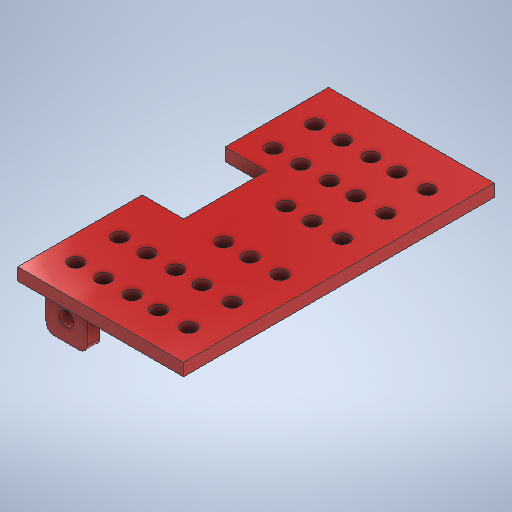
# Autodesk Inventor part: étage_servo
Saved by Autodesk Inventor 2025.1 (Build 291241000, 241)
## iProperties
Created: 2024-11-29
Part Number: étage_servo
Material: Générique
Document SubType Name: Modeling
Designer: yasmi
Density: 1 g/cm^3
Appearance: Par défaut
Author: yasmi
Autodesk Inventor part; units mm, degrees
ref_plane "YZ Plane" through (0, 0, 0) normal (1, 0, 0) x (0, 1, 0)
ref_plane "XZ Plane" through (0, 0, 0) normal (0, 1, 0) x (-1, 0, 0)
ref_plane "XY Plane" through (0, 0, 0) normal (0, 0, 1) x (1, 0, 0)
sketch "Esquisse1" plane through (0, 0, 0) normal (0, 1, 0) x (-1, 0, 0)
  line L0 (21.1354, -34.867) -> (21.1354, 40.133)
  circle A0 centre (1.447, -25.4161) radius 1.75
  circle A1 centre (1.447, -15.4161) radius 1.75
  circle A2 centre (8.3757, -15.4161) radius 1.75
  circle A3 centre (1.447, -4.8968) radius 1.75
  circle A4 centre (8.3757, -25.4161) radius 1.75
  line L1 (11.1354, 10.1032) -> (11.1354, -9.8968)
  line L2 (11.1354, -9.8968) -> (21.1354, -9.8968)
  line L3 (21.1354, -9.8968) -> (21.1354, 10.1032)
  line L4 (21.1354, 10.1032) -> (11.1354, -9.8968)
  line L5 (11.1354, 10.1032) -> (21.1354, -9.8968)
  line L6 (21.1354, 10.1032) -> (11.1354, 10.1032)
  line L7 (-18.8646, -34.867) -> (21.1354, -34.867)
  line L8 (-18.8646, -34.867) -> (21.1354, -34.867)
  line L9 (21.1354, -34.867) -> (21.1354, 40.133)
  line L10 (-18.8646, 40.133) -> (-18.8646, -34.867)
  line L11 (21.1354, 40.133) -> (-18.8646, 40.133)
  circle A5 centre (-68.4692, 33.6895) radius 1.75
  circle A6 centre (-68.4692, 42.6792) radius 1.75
  circle A7 centre (-4.9148, -25.4161) radius 1.75
  circle A8 centre (-4.9148, -15.4161) radius 1.75
  circle A9 centre (-4.9148, -4.8968) radius 1.75
  circle A10 centre (-12.188, -25.4161) radius 1.75
  circle A11 centre (-12.188, -15.4161) radius 1.75
  circle A12 centre (-12.188, -4.8968) radius 1.75
  circle A13 centre (15, -15.4161) radius 1.75
  circle A14 centre (15, -25.4161) radius 1.75
  circle A15 centre (1.447, 21.6987) radius 1.75
  circle A16 centre (1.447, 32.218) radius 1.75
  circle A17 centre (8.3757, 32.218) radius 1.75
  circle A18 centre (8.3757, 21.6987) radius 1.75
  circle A19 centre (-4.9148, 32.218) radius 1.75
  circle A20 centre (-4.9148, 21.6987) radius 1.75
  circle A21 centre (-12.188, 32.218) radius 1.75
  circle A22 centre (-12.188, 21.6987) radius 1.75
  circle A23 centre (15, 32.218) radius 1.75
  circle A24 centre (15, 21.6987) radius 1.75
  circle A25 centre (1.447, 10.1642) radius 1.75
  circle A26 centre (-4.9148, 10.1193) radius 1.75
  circle A27 centre (-12.188, 10.1193) radius 1.75
  point P0 (0, 0)
  point P1 (-36.8646, 0.1032)
  point P2 (-36.8646, 0.1032)
  point P3 (30.1354, 0.1032)
  point P4 (-36.8646, 0.1032)
  point P5 (16.1354, 0.1032)
  dimension "d28" = 40
  dimension "d30" = 75
  constraints: 28 centre point, 24 end point, 2 perpendicular, 1 coincident, 1 horizontal, 1 parallel
  measures "d28" distance of L7.start L8.end
  measures "d30" distance of L8.end L0.end
extrude "Extrusion1" add sketch "Esquisse1" along normal blind 3 contours L7 L10 L11 L0 L6 L1 L2
sketch "Esquisse2" plane through (0, 0, 0) normal (0, -1, 0) x (1, 0, 0)
  line L0 (18.8646, -34.867) -> (-21.1354, -34.867) projected
  line L1 (-21.1354, -34.867) -> (-21.1354, -9.8968) projected
  line L2 (-7.3354, -28.867) -> (-17.3354, -28.867)
  line L3 (-17.3354, -28.867) -> (-17.3354, -31.867)
  line L4 (-17.3354, -31.867) -> (-7.3354, -31.867)
  line L5 (-7.3354, -31.867) -> (-7.3354, -28.867)
  line L6 (-7.3354, -28.867) -> (-17.3354, -31.867) construction
  line L7 (-17.3354, -28.867) -> (-7.3354, -31.867) construction
  line L8 (-21.1354, 10.1032) -> (-21.1354, 40.133) projected
  line L9 (-21.1354, 40.133) -> (18.8646, 40.133) projected
  line L10 (-17.3354, 34.133) -> (-7.3354, 34.133)
  line L11 (-7.3354, 34.133) -> (-7.3354, 37.133)
  line L12 (-7.3354, 37.133) -> (-17.3354, 37.133)
  line L13 (-17.3354, 37.133) -> (-17.3354, 34.133)
  line L14 (-17.3354, 34.133) -> (-7.3354, 37.133) construction
  line L15 (-7.3354, 34.133) -> (-17.3354, 37.133) construction
  point P0 (0, 0)
  point P1 (-12.3354, -30.367)
  point P2 (-12.3354, 35.633)
  point P3 (-17.3354, -34.867)
  point P4 (-7.3354, -34.867)
  point P5 (-7.3354, 40.133)
  point P6 (-17.3354, 40.133)
  dimension "d34" = 8.8
  dimension "d35" = 4.5
  dimension "d36" = 10
  dimension "d37" = 3
  dimension "d38" = 8.8
  dimension "d39" = 4.5
  dimension "d40" = 10
  dimension "d41" = 3
  constraints: 24 end point, 4 midpoint, 4 parallel, 2 horizontal, 2 perpendicular
  measures "d34" distance from line of L1 point (-12.335, -30.367)
  measures "d35" distance from line of L0 point (-12.335, -30.367)
  measures "d36" distance of L4.end L3.end
  measures "d37" distance of L3.end L2.end
  measures "d38" distance from line of L8 point (-12.335, 35.633)
  measures "d39" distance from line of L9 point (-12.335, 35.633)
  measures "d40" distance of L12.end L11.end
  measures "d41" distance of L11.end L10.end
sketch "Esquisse4" plane through (-21.1354, 3, 40.133) normal (0, 0, 1) x (1, 0, 0)
  line L0 (10, -3) -> (0, -3) projected
  line L1 (13.8, -3) -> (13.8, -13) projected
  line L2 (3.7966, -3) -> (13.8, -13)
  line L3 (13.8, -13) -> (13.8, -3)
  line L4 (13.8, -3) -> (3.8, -13.0034)
  circle A0 centre (8.8, -8) radius 1.75 projected
  circle A1 centre (8.8, -8) radius 1.75
  point P0 (21.1354, -3)
  dimension "d48" = 3.5
  constraints: 6 end point, 1 centre point, 1 coincident, 1 collinear, 1 perpendicular, 1 point on line
  measures "d48" diameter of A1
extrude "Extrusion5" cut sketch "Esquisse4" against normal blind 3 contours A0 L2 L4 | L4 L2 A0 | A0 L4 L2 | L4 A0 L2
extrude "Extrusion6" add sketch "Esquisse2" along normal blind 10
sketch "Esquisse5" plane through (-7.3354, 0, -31.867) normal (0, 0, -1) x (-1, 0, 0)
  line L0 (0, -10) -> (10, 0)
  line L1 (10, 0) -> (10, -10)
  line L2 (0, 0) -> (0, -10) projected
  line L3 (10, -10) -> (0, 0)
  circle A0 centre (5, -5) radius 1.75
  point P0 (-7.3354, 0)
  dimension "d56" = 3.5
  constraints: 6 end point, 1 centre point, 1 midpoint, 1 perpendicular
  measures "d56" diameter of A0
extrude "Extrusion8" cut sketch "Esquisse5" against normal blind 3 contours A0 L3 L0 | L0 L3 A0 | L3 A0 L0 | L0 A0 L3
sketch "Esquisse6" plane through (-17.3354, 0, 37.133) normal (0, 0, 1) x (1, 0, 0)
  line L0 (10, -10) -> (0, 0)
  line L1 (6.2, 0) -> (-3.8, 0) projected
  line L2 (0, 0) -> (0, -10) projected
  line L3 (0, -10) -> (10, 0)
  line L4 (-3.8, 0) -> (36.2, 0) projected
  circle A0 centre (5, -5) radius 1.75
  point P0 (17.3354, 0)
  dimension "d61" = 3.5
  constraints: 4 end point, 2 point on line, 1 centre point, 1 midpoint, 1 perpendicular
  measures "d61" diameter of A0
extrude "Extrusion9" cut sketch "Esquisse6" against normal blind 3 contours A0 L3 L0 | L0 L3 A0 | L3 A0 L0 | L0 A0 L3
fillet "Congé3" radius 2 4 edges at (-17.3354, -10, 35.633) (-7.3354, -10, 35.633) (-17.3354, -10, -30.367) (-7.3354, -10, -30.367)
fillet "Congé4" radius 2 2 edges at (-17.3354, 0, -30.367) (-17.3354, 0, 35.633)
fillet "Congé5" radius 2 2 edges at (-7.3354, 0, -30.367) (-7.3354, 0, 35.633)
